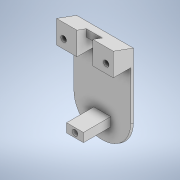
# Autodesk Inventor part: Ladesteckerhalter
Saved by Autodesk Inventor 2021 (Build 250183000, 183)
## iProperties
Created: 2024-06-24
Part Number: Ladesteckerhalter
Material: Generic
Document SubType Name: Modeling
Designer: Lukas
Density: 1 g/cm^3
Appearance: Default
Author: Lukas
Autodesk Inventor part; units mm, degrees
ref_plane "YZ Plane" through (0, 0, 0) normal (1, 0, 0) x (0, 1, 0)
ref_plane "XZ Plane" through (0, 0, 0) normal (0, 1, 0) x (-1, 0, 0)
ref_plane "XY Plane" through (0, 0, 0) normal (0, 0, 1) x (1, 0, 0)
sketch "Sketch1" plane through (0, 0, 0) normal (0, 0, 1) x (1, 0, 0)
  line L0 (-16, 6.5) -> (16, 6.5)
  line L1 (16, 6.5) -> (16, -6.5)
  line L2 (16, -6.5) -> (-16, -6.5)
  line L3 (-16, -6.5) -> (-16, 6.5)
  circle A0 centre (-12, -1.5) radius 1.6
  circle A1 centre (12, -1.5) radius 1.6
  point P0 (0, 0)
  point P1 (0, 6.5)
  point P2 (-16, 0)
  dimension "d0" = 32
  dimension "d1" = 13
  dimension "d2" = 12
  dimension "d3" = 24
  dimension "d4" = 5
  dimension "d5" = 3.2
  constraints: 8 end point, 2 centre point, 2 horizontal alignment, 2 midpoint, 2 parallel, 1 equal radius, 1 horizontal, 1 perpendicular, 1 vertical alignment
  measures "d0" distance of L0.start L0.end
  measures "d1" distance of L0.end L1.end
  measures "d2" horizontal distance of point (0, 0) A0.centre
  measures "d3" distance of A1.centre A0.centre
  measures "d4" distance from line of L2 A0.centre
  measures "d5" diameter of A0
extrude "Extrusion1" add sketch "Sketch1" along normal blind 9.8
sketch "Sketch2" plane through (0, 0, 9.8) normal (0, 0, 1) x (1, 0, 0)
  line L0 (-16, -6.5) -> (16, -6.5) projected
  line L1 (4.5, -6.5) -> (-4.5, -6.5)
  line L2 (-4.5, -6.5) -> (-4.5, 6.5)
  line L3 (16, 6.5) -> (-16, 6.5) projected
  line L4 (4.5, -6.5) -> (4.5, 6.5)
  point P0 (0, 0)
  point P1 (0, -6.5)
  point P2 (0, -6.5)
  point P3 (0, -6.5)
  dimension "d18" = 9
  constraints: 7 end point, 3 midpoint, 3 point on line, 2 perpendicular, 1 coincident, 1 horizontal, 1 vertical, 1 vertical alignment
  measures "d18" distance of L1.start L1.end
extrude "Extrusion2" cut sketch "Sketch2" against normal blind 5.25
chamfer "Chamfer1" distance 9.8 angle 20 1 edges at (0, 6.5, 0) measured on face at (0, 6.5, 0.5)
sketch "Sketch3" plane through (0, 0, 4.55) normal (0, 0, 1) x (1, 0, 0)
  line L0 (-4.5, -6.5) -> (-4.5, 4.5892) projected
  line L1 (4.5, 4.5892) -> (4.5, -6.5) projected
  line L2 (-4.5, -6.5) -> (4.5, -6.5)
  line L3 (4.5, -6.5) -> (4.5, 0.5)
  line L4 (4.5, 0.5) -> (-4.5, 0.5)
  line L5 (-4.5, 0.5) -> (-4.5, -6.5)
  point P0 (0, 0)
  point P1 (-4.5, 0.5)
  dimension "d19" = 7
  constraints: 8 end point, 2 parallel, 1 horizontal, 1 perpendicular, 1 point on line
  measures "d19" distance of L4.end L0.start
extrude "Extrusion4" cut sketch "Sketch3" against normal blind 4
sketch "Sketch5" plane through (-16, -6.5, 0) normal (-1, 0, 0) x (0, 0, 1)
  line L0 (0, 9.4331) -> (-1.5, 8.8871)
  line L1 (0, 9.4331) -> (9.8, 13) projected
  point P0 (0, 6.5)
  dimension "d28" = 1.5
  constraints: 2 end point, 1 collinear
  measures "d28" horizontal distance of L0.start L0.end
sketch "Sketch4" plane through (0, 0, 0) normal (0, 0, -1) x (-1, 0, 0)
  arc A0 (-15.9819, -32.9391) -> (16, -33.7) centre (0, -33.7) ccw
  line L0 (-16, -6.5) -> (-16, 6.5) projected
  line L1 (-16, -33.7) -> (-16, -6.5)
  line L2 (16, -33.7) -> (16, -6.5)
  line L3 (16, -6.5) -> (-16, -6.5) projected
  circle A1 centre (12, -1.5) radius 1.6 projected
  circle A2 centre (-12, -1.5) radius 1.6 projected
  line L4 (-16, 2.9331) -> (16, 2.9331) projected
  line L5 (-16, -6.5) -> (-16, 2.9331) projected
  line L6 (16, -6.5) -> (-16, -6.5) projected
  line L7 (16, 2.9331) -> (16, -6.5) projected
  circle A3 centre (0, -38.5) radius 1.6
  point P0 (0, 0)
  dimension "d22" = 27.2
  dimension "d23" = 3.2
  dimension "d25" = 37
  constraints: 4 end point, 3 point on circle, 2 centre point, 2 horizontal alignment, 2 tangent, 2 vertical, 1 coincident, 1 vertical alignment
  measures "d22" distance of L1.start L0.start
  measures "d23" diameter of A3
  measures "d25" vertical distance of A1.centre A3.centre
sketch3d "3D Sketch1"
sweep "Sweep1" add profiles "Sketch4" path "Sketch5" path curves L0 contours L1 L3 L2 A0 | L0 L4 L7 L3 | A1 | A2 | A3
extrude "Extrusion5" cut sketch "Sketch4" along normal through all contours A1 | A2 | A3
sketch "Sketch6" plane through (0, -33.7, 0) normal (0, 0, 1) x (1, 0, 0)
  line L0 (4.75, -7.3) -> (-4.75, -7.3)
  line L1 (-4.75, -7.3) -> (-4.75, -2.3)
  line L2 (-4.75, -2.3) -> (4.75, -2.3)
  line L3 (4.75, -2.3) -> (4.75, -7.3)
  circle A0 centre (0, -4.8) radius 1.6 projected
  point P0 (0, 33.7)
  point P1 (0, -7.3)
  point P2 (-4.75, -4.8)
  dimension "d31" = 5
  dimension "d32" = 9.5
  constraints: 8 end point, 2 midpoint, 2 parallel, 1 horizontal, 1 horizontal alignment, 1 perpendicular, 1 vertical alignment
  measures "d31" distance of L0.end L1.end
  measures "d32" distance of L1.end L2.end
extrude "Extrusion6" add sketch "Sketch6" along normal blind 15.4
sketch "Sketch7" plane through (-16, -34.246, -1.5) normal (0, 0, -1) x (-1, 0, 0)
  circle A0 centre (-16, 25.746) radius 1.4
  circle A1 centre (-16, -4.254) radius 1.6 projected
  point P0 (-16, 34.246)
  dimension "d35" = 30
  dimension "d36" = 2.8
  constraints: 1 centre point, 1 vertical alignment
  measures "d35" distance of A1.centre A0.centre
  measures "d36" diameter of A0
extrude "Extrusion7" cut sketch "Sketch7" against normal through all contours A0
equation "\"d2\" = 0.5 * d3"
body "Solid1"
